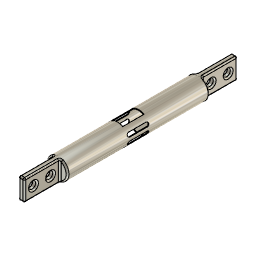
_Lower Leg.fc2c5f81-b364-426b-87a3-895b9db83cba (Autodesk Fusion 360 design; units mm, degrees)
Autodesk Fusion 360 part; units mm, degrees
note: some values were not read from the file. Chosen so that the rebuilt part matches the saved one: a direction. Set by a fixed rule: which sketch regions a step uses.
sketch "Sketch1" plane through (0, 0, 0) normal (0, 1, 0) x (1, 0, 0)
  line L0 (-4, 14.456832) -> (-4, -14.456832)
  circle A0 centre (0, 0) radius 14
  line L1 (4, 0) -> (-4, 0) construction
  circle A1 centre (0, 0) radius 15
  line L2 (4, 14.456832) -> (4, -14.456832)
  dimension "d413" = 30
  dimension "d414" = 28
  dimension "d419" = 8
  constraint concentric A0 A1
  constraint vertical L0
  constraint parallel L0 L2
  constraint midpoint L1.start L2
  constraint midpoint L1.end L0
  constraint midpoint A0.centre L1
  constraint coincident A0.centre A1.centre
  measures "d413" diameter of A1
  measures "d414" diameter of A0
  measures "d419" distance of L1.end L1.start
extrude "Extrude1" add sketch "Sketch1" along normal blind 2
extrude "Extrude2" add sketch "Sketch1" along normal blind 100 contours L0 A0 A1 L2 | L0 A0 A1 | A0 A1 L2 | L0 A0 A1 L2 picked at (3.340391, 13.908858) picked at (-4.680206, -13.867723) picked at (4.680206, -13.867723) picked at (3.340391, -13.908858)
extrude "Extrude3" add sketch "Sketch1" against normal blind 50 contours L0 A0 A1 L2 | L0 A0 L2 | L0 A0 A1 L2 picked at (3.340391, 13.908858) picked at (-1.333333, 4.472136) picked at (3.340391, -13.908858)
sketch "Sketch2" plane through (4, 0, 0) normal (1, 0, 0) x (0, 1, 0)
  line L0 (0, -14.456832) -> (0, 14.456832)
  line L1 (0, 14.456832) -> (-50, 14.456832)
  line L2 (-50, 14.456832) -> (-50, -14.456832)
  line L3 (-50, -14.456832) -> (0, -14.456832)
  line L4 (-50, -14.456832) -> (0, -14.456832)
  line L5 (-37, 0) -> (-25, 0) construction
  circle A0 centre (-13, 0) radius 5
  line L6 (-50, 14.456832) -> (-50, -14.456832)
  circle A1 centre (-37, 0) radius 5
  line L7 (-25, 0) -> (-13, 0) construction
  line L8 (-25, 14.456832) -> (-25, -14.456832) construction
  line L9 (0, 14.456832) -> (-50, 14.456832)
  line L10 (0, -14.456832) -> (0, 14.456832)
  point P0 (0.432473, -42.490513)
  dimension "d431" = 10
  dimension "d491" = 10
  dimension "d538" = 24
  constraint horizontal L5.start A0.centre
  constraint coincident L5.start A1.centre
  constraint midpoint L5.end L8
  constraint perpendicular L5 L8
  constraint coincident A0.centre L7.end
  constraint perpendicular L7 L8
  constraint equal L5 L7
  constraint vertical L6
  constraint horizontal L4
  constraint vertical L10
  constraint horizontal L9
  measures "d431" diameter of A0
  measures "d491" diameter of A1
  measures "d538" distance of L5.start A0.centre
extrude "Extrude4" cut sketch "Sketch2" against normal blind 8 contours A0 | A1 picked at (-14.626165, 0.938867) picked at (-38.286058, 0.706986)
fillet "Fillet1" radius 2 5 faces at (9.053609, 0, 3.307068) (4, -28.391098, -11.189344) (0.672785, -50, 4.954529) (-4, -28.391098, -11.189344) (-7.777185, 0, 3.307068)
mirror "Mirror1" about plane through (0, 100, 0) normal (0, 1, 0) of bodies 1 merged
sketch "Sketch3" plane through (0, 0, 0) normal (0, 0, -1) x (0, 1, 0)
  line L0 (115, 7.5) -> (85, 7.5)
  line L1 (85, 7.5) -> (85, -7.5)
  line L2 (85, -7.5) -> (115, -7.5)
  line L3 (115, -7.5) -> (115, 7.5)
  line L4 (115, 7.5) -> (85, -7.5) construction
  line L5 (85, 7.5) -> (115, -7.5) construction
  circle A0 centre (-13, 0) radius 5 construction
  circle A1 centre (213, 0) radius 5 construction
  line L6 (-13, 0) -> (213, 0) construction
  point P0 (100, 0)
  dimension "d20" = 30
  dimension "d21" = 15
  constraint horizontal L0
  constraint perpendicular L0 L1
  constraint parallel L0 L2
  constraint parallel L1 L3
  constraint coincident L4 P0
  constraint coincident L5 P0
  constraint coincident A0.centre L6.start
  constraint coincident A1.centre L6.end
  constraint midpoint P0 L6
  measures "d20" distance of L1.end L2.end
  measures "d21" distance of L0.end L1.end
extrude "Extrude5" cut sketch "Sketch3" along normal mid plane 40
sketch "Sketch4" plane through (0, 0, 0) normal (1, 0, 0) x (0, 0, -1)
  circle A0 centre (5, 87.5) radius 2.5
  circle A1 centre (-5, 87.5) radius 2.5
  line L0 (-5, 87.5) -> (5, 87.5) construction
  line L1 (-2.307692, 248) -> (2.307692, 248)
  line L2 (-2.307692, -48) -> (2.307692, -48)
  line L3 (0, 248) -> (0, -48) construction
  circle A2 centre (5, 112.5) radius 2.5
  circle A3 centre (-5, 112.5) radius 2.5
  line L4 (-5, 112.5) -> (5, 112.5) construction
  line L5 (0, 87.5) -> (0, 112.5)
  line L6 (7.5, 87.5) -> (7.5, 112.5)
  line L7 (-7.5, 112.499956) -> (-7.5, 87.5)
  line L8 (-2.5, 87.5) -> (-2.5, 112.5)
  line L9 (2.5, 112.5) -> (2.5, 87.5)
  point P0 (7.5, 85)
  point P1 (0, 87.5)
  point P2 (0, 112.5)
  dimension "d24" = 5
  dimension "d25" = 5
  dimension "d26" = 10
  dimension "d29" = 5
  dimension "d30" = 5
  dimension "d31" = 10
  dimension "d33" = 25
  constraint coincident A1.centre L0.start
  constraint coincident A0.centre L0.end
  constraint horizontal L0
  constraint midpoint L1 L3.start
  constraint midpoint L2 L3.end
  constraint midpoint L0 P1
  constraint coincident L3 P1
  constraint coincident A3.centre L4.start
  constraint coincident A2.centre L4.end
  constraint horizontal L4
  constraint midpoint L4 P2
  constraint coincident L3 P2
  constraint coincident P1 L5.start
  constraint coincident P2 L5.end
  constraint midpoint L3 L5
  constraint coincident A0 L6.start
  constraint coincident A2 L6.end
  constraint tangent A2 L6
  constraint coincident A1 L7.end
  constraint tangent A1 L7
  constraint parallel L3 L7
  constraint coincident L0 L8.start
  constraint coincident A1 L8.start
  constraint coincident A3 L8.end
  constraint tangent A3 L8
  constraint coincident L4 L9.start
  constraint coincident A2 L9.start
  constraint coincident A0 L9.end
  constraint coincident L0 L9.end
  constraint tangent A0 L6
  measures "d24" diameter of A0
  measures "d25" diameter of A1
  measures "d26" distance of A1.centre A0.centre
  measures "d29" diameter of A2
  measures "d30" diameter of A3
  measures "d31" distance of A3.centre A2.centre
  measures "d33" distance of P1 P2
extrude "Extrude6" cut sketch "Sketch4" along normal mid plane 40
